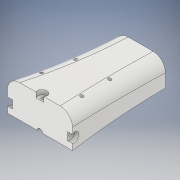
# Autodesk Inventor part: AA008
Saved by Autodesk Inventor 2017 SP1 (Build 210196100, 196)
## iProperties
Created: 2017-09-28
Part Number: AA008
Material: ABS Plastic
Document SubType Name: Modeling
Designer: Zach
Density: 1.06 g/cm^3
Appearance: CR White
Author: Zach
Autodesk Inventor part; units mm, degrees
sketch "Sketch1" plane through (0, 0, 0) normal (0, 0, 1) x (1, 0, 0)
  line L0 (0, 0) -> (80, 0)
  line L1 (80, 0) -> (80, 82.6)
  line L2 (80, 82.6) -> (0, 82.6)
  line L3 (0, 82.6) -> (0, 0)
  dimension "d0" = 80
  dimension "d1" = 82.6
  constraints: 8 end point, 2 parallel, 1 horizontal, 1 perpendicular
  measures "d0" distance of L2.end L1.end
  measures "d1" distance of L1.end L0.end
extrude "Extrusion1" add sketch "Sketch1" along normal blind 162.5
sketch "Sketch2" plane through (0, 82.6, 0) normal (0, 1, 0) x (1, 0, 0)
  line L0 (0, -162.5) -> (80, -162.5) projected
  line L1 (-12.5, -162.5) -> (0, -162.5)
  line L2 (80, -162.5) -> (92.5, -162.5)
  line L3 (0, 0) -> (80, 0) projected
  line L4 (0, 0) -> (0, -162.5) projected
  line L5 (80, 0) -> (80, -162.5) projected
  arc A0 (-12.5, -162.5) -> (0, 0) centre (-1199.9534, 10.5733) ccw
  arc A1 (80, 0) -> (92.5, -162.5) centre (1279.9534, 10.5733) ccw
  dimension "d4" = 12.5
  dimension "d5" = 12.5
  dimension "d19" = 1200
  dimension "d20" = 1200
  constraints: 4 end point, 4 point on circle, 2 centre point, 1 collinear, 1 parallel
  measures "d4" distance of L1.start L0.start
  measures "d5" distance of L0.end L2.end
  measures "d19" radius of A0
  measures "d20" radius of A1
extrude "Extrusion2" add sketch "Sketch2" against normal blind 82.6 contours L1 A0 L4 | L5 A1 L2
sketch "Sketch5" plane through (0, 0, 0) normal (0, 0, -1) x (-1, 0, 0)
  line L0 (12.5, 0) -> (-92.5, 0)
  line L1 (-92.5, 0) -> (-92.5, 41.3)
  line L2 (-92.5, 41.3) -> (12.5, 41.3)
  line L3 (12.5, 41.3) -> (12.5, 0)
  point P0 (0, 0)
  point P1 (12.5, 20)
  point P2 (-92.5, 20)
  dimension "d22" = 41.3
  constraints: 8 end point, 2 parallel, 2 point on line, 1 horizontal, 1 horizontal alignment, 1 perpendicular
  measures "d22" distance of L0.end L1.end
extrude "Extrusion4" cut sketch "Sketch5" against normal through all
sketch "Sketch8" plane through (0, 0, 0) normal (1, 0, 0) x (0, 1, 0)
  line L0 (82.6, 162.5) -> (93.8, 162.5)
  line L1 (41.3, 162.5) -> (41.3, 0) projected
  line L2 (82.6, 0) -> (41.3, 0) projected
  arc A0 (93.8, 162.5) -> (82.6, 0) centre (2580.9593, -90.5586) ccw
  line L3 (82.6, 162.5) -> (41.3, 162.5) projected
  line L4 (82.6, 162.5) -> (82.6, 0)
  point P0 (0, 0)
  dimension "d32" = 2500
  dimension "d38" = 11.2
  constraints: 4 end point, 2 point on circle, 1 centre point, 1 horizontal, 1 perpendicular
  measures "d32" radius of A0
  measures "d38" distance of L0.start L0.end
extrude "Extrusion6" add sketch "Sketch8" along normal blind 93 and the other way blind 13 contours L0 A0 L4
sketch "Sketch13" plane through (-13, 82.6, 0) normal (0, -1, 0) x (1, 0, 0)
  arc A0 (13, 0) -> (0.5, 162.5) centre (-1186.9534, -10.5733) ccw projected
  line L0 (0, 162.5) -> (0.5, 162.5) projected
  line L1 (0, 0) -> (0, 162.5) projected
  line L2 (13, 0) -> (0, 0) projected
  arc A1 (105.5, 162.5) -> (93, 0) centre (1292.9534, -10.5733) ccw projected
  line L3 (106, 0) -> (93, 0) projected
  line L4 (106, 162.5) -> (106, 0) projected
  line L5 (105.5, 162.5) -> (106, 162.5) projected
  point P0 (13, 0)
extrude "Extrusion9" cut sketch "Sketch13" against normal through all
fillet "Fillet4" radius 20 2 edges at (-3.5176, 86.9111, 81.8462) (83.5176, 86.9111, 81.8462)
ref_plane "Work Plane5" through (72.5841, 93.8, 162.5) normal (0, 1, 0) x (-1, 0, 0)
sketch "Sketch27" plane through (72.5841, 93.8, 162.5) normal (0, 1, 0) x (-1, 0, 0)
  line L0 (65.1681, 0) -> (0, 0)
  line L1 (-4.9159, 0) -> (70.0841, 0)
  circle A0 centre (32.5841, -4) radius 7.5
  point P0 (72.5841, -162.5)
  point P1 (32.5841, 0)
  dimension "d91" = 15
  dimension "d94" = 4
  constraints: 4 end point, 1 centre point, 1 midpoint, 1 vertical alignment
  measures "d91" diameter of A0
  measures "d94" distance of point (32.584, 0) A0.centre
extrude "Extrusion19" cut sketch "Sketch27" against normal blind 8
sketch "Sketch29" plane through (72.5841, 85.8, 162.5) normal (0, 1, 0) x (1, 0, 0)
  circle A0 centre (-32.5841, 4) radius 2
  arc A1 (-26.2398, 0) -> (-38.9284, 0) centre (-32.5841, 4) ccw projected
  point P0 (-72.5841, 162.5)
  dimension "d95" = 4
  constraints: 1 centre point, 1 concentric, 1 horizontal alignment
  measures "d95" diameter of A0
extrude "Extrusion20" cut sketch "Sketch29" against normal through all
ref_plane "Work Plane6" through (-12.5, 41.3, 162.5) normal (1, 0, 0) x (0, 1, 0)
sketch "Sketch30" plane through (-12.5, 41.3, 162.5) normal (1, 0, 0) x (0, 1, 0)
  line L0 (32.6904, 0) -> (0, 0) projected
  circle A0 centre (16.3452, -4) radius 7.5
  point P0 (-41.3, -162.5)
  point P1 (16.3452, 0)
  dimension "d98" = 15
  dimension "d99" = 4
  constraints: 1 centre point, 1 midpoint, 1 vertical alignment
  measures "d98" diameter of A0
  measures "d99" distance from line of L0 A0.centre
extrude "Extrusion21" cut sketch "Sketch30" along normal blind 8
sketch "Sketch32" plane through (-4.5, 41.3, 162.5) normal (-1, 0, 0) x (0, 0, 1)
  circle A0 centre (-4, 16.3452) radius 2
  arc A1 (0, 22.6895) -> (0, 10.0009) centre (-4, 16.3452) ccw projected
  point P0 (-162.5, -41.3)
  dimension "d102" = 4
  constraints: 1 centre point, 1 concentric, 1 vertical alignment
  measures "d102" diameter of A0
extrude "Extrusion22" cut sketch "Sketch32" against normal through all
ref_plane "Work Plane7" through (92.5, 41.3, 162.5) normal (1, 0, 0) x (0, 1, 0)
sketch "Sketch33" plane through (92.5, 41.3, 162.5) normal (1, 0, 0) x (0, 1, 0)
  spline S0 degree 7 poles (16.3452, -2) (16.5842, -2) (16.823, -2.0333) (17.0589, -2.0999) (17.2885, -2.2007) (17.5074, -2.3374) (17.7098, -2.5118) (18.0398, -2.9108) (18.1792, -3.1324) (18.2884, -3.3855) (18.3565, -3.661) (18.3776, -3.9466) (18.3512, -4.2293) (18.2119, -4.7719) (18.0994, -5.0216) (17.9544, -5.2419) (17.785, -5.431) (17.5982, -5.5882) (17.4002, -5.7139) (16.9472, -5.9271) (16.6861, -6.0009) (16.4192, -6.0336) (16.1506, -6.0259) (15.8845, -5.9774) (15.6259, -5.8869) (15.1979, -5.6516) (15.02, -5.5245) (14.853, -5.3705) (14.7022, -5.1893) (14.5734, -4.9818) (14.4729, -4.75) (14.3444, -4.2496) (14.3167, -3.9882) (14.3298, -3.7231) (14.3837, -3.465) (14.4743, -3.2243) (14.5929, -3.0092) (14.9036, -2.5816) (15.1129, -2.383) (15.3429, -2.2275) (15.586, -2.1131) (15.8367, -2.0377) (16.0909, -2) (16.3452, -2) knots 0 0 0 0 0 0 0 0 0.152749 0.152749 0.152749 0.152749 0.152749 0.152749 0.285714 0.285714 0.285714 0.285714 0.285714 0.285714 0.421907 0.421907 0.421907 0.421907 0.421907 0.421907 0.58891 0.58891 0.58891 0.58891 0.58891 0.58891 0.71461 0.71461 0.71461 0.71461 0.71461 0.71461 0.837939 0.837939 0.837939 0.837939 0.837939 0.837939 1 1 1 1 1 1 1 1 projected
  circle A0 centre (16.3452, -4) radius 2 projected
  circle A1 centre (16.3452, -4) radius 7.5
  point P0 (-41.3, -162.5)
  dimension "d105" = 15
  constraints: 1 centre point, 1 coincident, 1 vertical alignment, 1 other
  measures "d105" diameter of A1
extrude "Extrusion23" cut sketch "Sketch33" against normal blind 8
sketch "Sketch38" plane through (0, 0, 162.5) normal (0, 0, 1) x (1, 0, 0)
  line L0 (75, 41.3) -> (5, 41.3)
  circle A0 centre (40, 41.3) radius 4.5
  point P0 (0, 0)
  dimension "d117" = 9
  constraints: 2 end point, 1 centre point, 1 midpoint
  measures "d117" diameter of A0
extrude "Extrusion27" cut sketch "Sketch38" against normal through all
ref_plane "Work Plane14" through (0, 0, 152.5) normal (0, 0, 1) x (1, 0, 0)
sketch "Sketch40" plane through (0, 0, 152.5) normal (0, 0, 1) x (1, 0, 0)
  arc A0 (44.5, 41.3) -> (35.5, 41.3) centre (40, 41.3) ccw projected
  circle A1 centre (40, 41.3) radius 11.5
  point P0 (0, 0)
  dimension "d121" = 23
  constraints: 1 centre point, 1 coincident
  measures "d121" diameter of A1
extrude "Extrusion28" cut sketch "Sketch40" against normal blind 9
ref_plane "Work Plane15" through (0, 0, 61.5) normal (0, 0, 1) x (1, 0, 0)
sketch "Sketch41" plane through (0, 0, 61.5) normal (0, 0, 1) x (1, 0, 0)
  arc A0 (44.5, 41.3) -> (35.5, 41.3) centre (40, 41.3) ccw
  circle A1 centre (40, 41.3) radius 11.5
  point P0 (0, 0)
  dimension "d125" = 23
  constraints: 2 centre point, 2 point on circle, 1 coincident
  measures "d125" diameter of A1
extrude "Extrusion29" cut sketch "Sketch41" against normal blind 9
ref_plane "Work Plane16" through (0, 0, 47.5) normal (0, 0, 1) x (1, 0, 0)
sketch "Sketch43" plane through (0, 0, 47.5) normal (0, 0, 1) x (1, 0, 0)
  arc A0 (44.5, 41.3) -> (35.5, 41.3) centre (40, 41.3) ccw
  line L0 (35.5, 41.3) -> (0, 41.3) construction
  line L1 (0, 62.5933) -> (0, 41.3) construction
  spline S0 degree 3 poles (19.9943, 82.6) (17.3915, 82.6) (14.8137, 82.0916) (9.998, 80.1152) (7.8062, 78.6662) (4.1001, 75.0086) (2.6216, 72.8347) (1.0742, 69.2017) (0.6732, 67.9146) (0.1355, 65.2795) (0, 63.9381) (0, 62.5933) knots 0 0 0 0 0.78083 0.78083 1.561665 1.561665 2.342928 2.342928 2.746314 2.746314 3.149743 3.149743 3.149743 3.149743 construction
  line L2 (60.0057, 82.6) -> (19.9943, 82.6) construction
  spline S1 degree 3 poles (80, 62.5933) (80, 65.2007) (79.4908, 67.7832) (77.5113, 72.6059) (76.0606, 74.8001) (72.4005, 78.5072) (70.2269, 79.985) (66.5969, 81.5295) (65.3131, 81.9291) (62.6848, 82.465) (61.3469, 82.6) (60.0057, 82.6) knots 0 0 0 0 0.782215 0.782215 1.563936 1.563936 2.345071 2.345071 2.747441 2.747441 3.149817 3.149817 3.149817 3.149817 construction
  line L3 (80, 41.3) -> (80, 62.5933) construction
  line L4 (80, 41.3) -> (44.5, 41.3) construction
  line L5 (60.0057, 80.6) -> (19.9943, 80.6)
  line L6 (2, 62.5933) -> (2, 43.3)
  line L7 (2, 43.3) -> (33.8153, 43.3) construction
  arc A1 (46.1847, 43.3) -> (33.8153, 43.3) centre (40, 41.3) ccw construction
  line L8 (46.1847, 43.3) -> (78, 43.3) construction
  line L9 (78, 43.3) -> (78, 62.5933)
  line L10 (2, 43.3) -> (2, 41.3)
  line L11 (78, 43.3) -> (78, 41.3)
  line L12 (44.5, 41.3) -> (78, 41.3)
  line L13 (35.5, 41.3) -> (2, 41.3)
  line L14 (5, 41.3) -> (35.5, 41.3)
  arc A2 (44.5, 41.3) -> (35.5, 41.3) centre (40, 41.3) ccw projected
  spline S2 degree 5 poles (78, 62.5933) (77.9999, 65.4195) (77.4463, 68.2457) (76.3377, 70.927) (73.1281, 75.7135) (68.3466, 78.931) (65.6637, 80.0441) (62.8346, 80.5999) (60.0057, 80.6) knots 0 0 0 0 0 0 0.499755 0.499755 0.499755 1 1 1 1 1 1
  spline S3 degree 5 poles (19.9943, 80.6) (17.1686, 80.5999) (14.3427, 80.0454) (11.6625, 78.9348) (6.8791, 75.7206) (3.666, 70.9361) (2.5549, 68.2521) (2.0001, 65.4227) (2, 62.5933) knots 0 0 0 0 0 0 0.499678 0.499678 0.499678 1 1 1 1 1 1
  dimension "d129" = 2
  constraints: 30 end point, 4 point on circle, 3 centre point, 3 parallel, 2 perpendicular, 2 point on line, 1 collinear, 1 horizontal, 1 horizontal alignment, 18 other
  measures "d129" distance between parallel lines of L3 L9
extrude "Extrusion30" cut sketch "Sketch43" against normal blind 35
sketch "Sketch53" plane through (0, 0, 12.5) normal (0, 0, 1) x (1, 0, 0)
  arc A0 (44.5, 41.3) -> (35.5, 41.3) centre (40, 41.3) ccw projected
  circle A1 centre (40, 41.3) radius 2.5 construction
  line L0 (44.5, 41.3) -> (42.5, 41.3)
  line L1 (35.5, 41.3) -> (37.5, 41.3)
  arc A2 (42.5, 41.3) -> (37.5, 41.3) centre (40, 41.3) ccw
  point P0 (0, 0)
  dimension "d163" = 5
  constraints: 4 end point, 4 point on circle, 2 centre point, 1 coincident, 1 concentric, 1 horizontal, 1 point on line
  measures "d163" diameter of A1
extrude "Extrusion39" add sketch "Sketch53" against normal blind 2
sketch "Sketch54" plane through (0, 0, 0) normal (0, 0, -1) x (-1, 0, 0)
  arc A0 (-35.5, 41.3) -> (-44.5, 41.3) centre (-40, 41.3) ccw projected
  circle A1 centre (-40, 41.3) radius 16.5
  point P0 (0, 0)
  dimension "d166" = 33
  constraints: 1 centre point, 1 coincident
  measures "d166" diameter of A1
extrude "Extrusion40" cut sketch "Sketch54" against normal blind 7.5
sketch "Sketch55" plane through (0, 0, 12.5) normal (0, 0, 1) x (1, 0, 0)
  arc A0 (42.5, 41.3) -> (37.5, 41.3) centre (40, 41.3) ccw projected
  circle A1 centre (40, 49.8) radius 2
  point P0 (0, 0)
  dimension "d169" = 4
  dimension "d170" = 8.5
  constraints: 1 centre point, 1 vertical alignment
  measures "d169" diameter of A1
  measures "d170" distance of A0.centre A1.centre
extrude "Extrusion41" cut sketch "Sketch55" against normal through all
sketch "Sketch56" plane through (0, 0, 12.5) normal (0, 0, 1) x (1, 0, 0)
  circle A0 centre (40, 49.8) radius 2 projected
  circle A1 centre (40, 49.8) radius 3.5
  point P0 (0, 0)
  dimension "d173" = 7
  constraints: 1 centre point, 1 coincident
  measures "d173" diameter of A1
extrude "Extrusion42" cut sketch "Sketch56" against normal blind 3
sketch "Sketch57" plane through (0, 0, 12.5) normal (0, 0, 1) x (1, 0, 0)
  arc A0 (42.5, 41.3) -> (37.5, 41.3) centre (40, 41.3) ccw construction
  line L0 (40, 41.3) -> (52.5, 62.9506) construction
  line L1 (52.5, 62.9506) -> (27.5, 62.9506) construction
  line L2 (27.5, 62.9506) -> (40, 41.3) construction
  circle A1 centre (52.5, 62.9506) radius 1.625
  circle A2 centre (27.5, 62.9506) radius 1.625
  point P0 (0, 0)
  dimension "d176" = 25
  dimension "d177" = 25
  dimension "d178" = 25
  dimension "d179" = 3.25
  dimension "d180" = 3.25
  constraints: 6 end point, 2 centre point, 2 coincident, 1 horizontal
  measures "d176" distance of L0.start L0.end
  measures "d177" distance of L0.end L1.end
  measures "d178" distance of L1.end L0.start
  measures "d179" diameter of A1
  measures "d180" diameter of A2
extrude "Extrusion43" cut sketch "Sketch57" along normal blind 50 and the other way blind 50
sketch "Sketch58" plane through (44.5, 41.3, 162.5) normal (0, -1, 0) x (1, 0, 0)
  line L0 (0, -19) -> (0, -101) construction
  line L1 (23, -85) -> (-32, -85) construction
  line L2 (28, -35) -> (-37, -35) construction
  line L3 (-9, -10) -> (0, -10) construction
  circle A0 centre (23, -85) radius 2.5
  circle A1 centre (-32, -85) radius 2.5
  circle A2 centre (-37, -35) radius 2.5
  circle A3 centre (28, -35) radius 2.5
  line L4 (-4.5, -35) -> (-4.5, -85) construction
  point P0 (-44.5, -162.5)
  point P1 (-4.5, -10)
  point P2 (-4.5, -60)
  point P3 (0, -60)
  dimension "d185" = 55
  dimension "d186" = 65
  dimension "d187" = 5
  dimension "d188" = 5
  dimension "d189" = 5
  dimension "d190" = 5
  dimension "d198" = 50
  constraints: 6 end point, 5 midpoint, 4 centre point, 4 coincident, 2 horizontal, 2 vertical alignment, 1 horizontal alignment, 1 vertical
  measures "d185" distance of L1.start L1.end
  measures "d186" distance of L2.start L2.end
  measures "d187" diameter of A0
  measures "d188" diameter of A1
  measures "d189" diameter of A2
  measures "d190" diameter of A3
  measures "d198" distance between parallel lines of L1 L2
extrude "Extrusion44" cut sketch "Sketch58" against normal through all
sketch "Sketch59" plane through (0, 0, 12.5) normal (0, 0, 1) x (1, 0, 0)
  arc A0 (42.5, 41.3) -> (37.5, 41.3) centre (40, 41.3) ccw construction
  circle A1 centre (52.5, 62.9506) radius 1.625 construction
  circle A2 centre (40, 41.3) radius 13.5 construction
  circle A3 centre (52.5, 62.9506) radius 13.5 construction
  circle A4 centre (27.5, 62.9506) radius 1.625 projected
  circle A5 centre (27.5, 62.9506) radius 7.5
  point P0 (0, 0)
  dimension "d193" = 27
  dimension "d194" = 27
  dimension "d195" = 15
  constraints: 3 centre point, 3 coincident
  measures "d193" diameter of A2
  measures "d194" diameter of A3
  measures "d195" diameter of A5
extrude "Extrusion45" add sketch "Sketch59" along normal blind 5
sketch "Sketch60" plane through (0, 0, 7.5) normal (0, 0, -1) x (-1, 0, 0)
  circle A0 centre (-40, 49.8) radius 2 projected
  line L0 (-23.5, 41.3) -> (-35.5, 41.3) projected
  arc A1 (-23.5, 41.3) -> (-56.5, 41.3) centre (-40, 41.3) ccw projected
  line L1 (-44.5, 41.3) -> (-56.5, 41.3) projected
  arc A2 (-35.5, 41.3) -> (-44.5, 41.3) centre (-40, 41.3) ccw projected
  arc A3 (-35.5, 41.3) -> (-44.5, 41.3) centre (-40, 41.3) ccw projected
  line L2 (-44.5, 41.3) -> (-42.5, 41.3) projected
  arc A4 (-37.5, 41.3) -> (-42.5, 41.3) centre (-40, 41.3) ccw projected
  line L3 (-37.5, 41.3) -> (-35.5, 41.3) projected
  circle A5 centre (-40, 41.3) radius 4.5
  circle A6 centre (-40, 41.3) radius 16.5
  circle A7 centre (-40, 32.8) radius 2
  point P0 (0, 0)
  dimension "d199" = 4
  constraints: 2 coincident, 2 horizontal alignment, 1 centre point, 1 symmetric about line, 4 other
  measures "d199" diameter of A7
extrude "Extrusion46" add sketch "Sketch60" against normal blind 5 contours A6 L1 A5 L0
sketch "Sketch61" plane through (0, 0, 10.5) normal (0, 0, -1) x (-1, 0, 0)
  circle A0 centre (-40, 41.3) radius 4.5 projected
  arc A1 (-37.5, 41.3) -> (-42.5, 41.3) centre (-40, 41.3) ccw projected
  line L0 (-37.5, 41.3) -> (-35.5, 41.3) projected
  circle A2 centre (-40, 41.3) radius 2.5
  point P0 (0, 0)
  constraints: 2 horizontal alignment, 1 coincident, 2 other
extrude "Extrusion47" add sketch "Sketch61" against normal blind 2
sketch "Sketch62" plane through (0, 0, 12.5) normal (0, 0, 1) x (1, 0, 0)
  circle A0 centre (40, 32.8) radius 2 projected
  circle A1 centre (40, 32.8) radius 3.5
  point P0 (0, 0)
  dimension "d204" = 7
  constraints: 1 centre point, 1 coincident
  measures "d204" diameter of A1
extrude "Extrusion48" cut sketch "Sketch62" against normal blind 3
equation "\"d5\" = d4"
body "Solid1"
